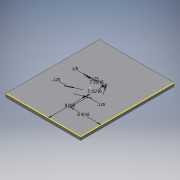
# Autodesk Inventor part: support platforms (for assembly)
Saved by Autodesk Inventor 2016 (Build 200138000, 138)
## iProperties
Created: 2017-10-23
Part Number: support platforms (for assembly)
Material: Generic
Document SubType Name: Modeling
Designer: student
Density: 1 g/cm^3
Appearance: Default
Author: student
Autodesk Inventor part; units mm, degrees
ref_plane "YZ Plane" through (0, 0, 0) normal (1, 0, 0) x (0, 1, 0)
ref_plane "XZ Plane" through (0, 0, 0) normal (0, 1, 0) x (-1, 0, 0)
ref_plane "XY Plane" through (0, 0, 0) normal (0, 0, 1) x (1, 0, 0)
sketch "Sketch1" plane through (0, 0, 0) normal (0, 1, 0) x (-1, 0, 0)
  line L0 (-203.2, 254) -> (203.2, 254)
  line L1 (203.2, 254) -> (203.2, -254)
  line L2 (203.2, -254) -> (-203.2, -254)
  line L3 (-203.2, -254) -> (-203.2, 254)
  line L4 (-203.2, 254) -> (203.2, -254) construction
  line L5 (203.2, 254) -> (-203.2, -254) construction
  point P0 (0, 0)
  dimension "d0" = 406.4
  dimension "d1" = 508
  constraints: 12 end point, 2 midpoint, 2 parallel, 1 horizontal, 1 perpendicular
  measures "d0" distance of L1.end L2.end
  measures "d1" distance of L0.end L1.end
extrude "Extrusion1" add sketch "Sketch1" along normal blind 19.05
sketch "Sketch2" plane through (0, 19.05, 0) normal (0, 1, 0) x (1, 0, 0)
  circle A0 centre (36.5125, -50.8) radius 1.5875
  circle A1 centre (-63.5, -50.8) radius 1.5875
  circle A2 centre (36.5125, 49.2125) radius 1.5875
  circle A3 centre (-63.5, 49.2125) radius 1.5875
  line L0 (203.2, -254) -> (203.2, 254) projected
  line L1 (203.2, -254) -> (-203.2, -254) projected
  point P0 (0, 0)
  dimension "d4" = 166.6875
  dimension "d5" = 203.2
  dimension "d6" = 100.0125
  dimension "d7" = 100.0125
  dimension "d9" = 3.175
  dimension "d10" = 3.175
  dimension "d11" = 3.175
  dimension "d12" = 3.175
  constraints: 4 centre point, 2 horizontal alignment, 2 vertical alignment
  measures "d4" distance from line of L0 A0.centre
  measures "d5" distance from line of L1 A0.centre
  measures "d6" distance of A0.centre A2.centre
  measures "d7" distance of A2.centre A3.centre
  measures "d9" diameter of A1
  measures "d10" diameter of A3
  measures "d11" diameter of A2
  measures "d12" diameter of A0
body "Solid1"
